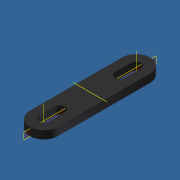
# Autodesk Inventor part: clamp
Saved by Autodesk Inventor 2014 SP2 (Build 180246200, 246)
## iProperties
Created: 2015-02-01
Part Number: clamp
Material: ABS-Kunststoff - Schwarz
Document SubType Name: Modeling
Designer: 4ndreas
Density: 1.06 g/cm^3
Appearance: Glatt - weiß(2)
Author: 4ndreas
Autodesk Inventor part; units mm, degrees
ref_plane "YZ Plane" through (0, 0, 0) normal (1, 0, 0) x (0, 1, 0)
ref_plane "XZ Plane" through (0, 0, 0) normal (0, 1, 0) x (-1, 0, 0)
ref_plane "XY Plane" through (0, 0, 0) normal (0, 0, 1) x (1, 0, 0)
sketch "Skizze1" plane through (0, 0, 0) normal (0, 0, 1) x (1, 0, 0)
  arc A0 (-9.8094, 24.1784) -> (-25.5, 32.4636) centre (-25.5, 13.4636) ccw projected
  spline S0 degree 3 poles (-9.5246, 24.4295) (-9.5947, 24.3508) (-9.6913, 24.2673) (-9.8094, 24.1784) knots -3.5231 -3.5231 -3.5231 -3.5231 -3.387334 -3.387334 -3.387334 -3.387334 projected
  spline S1 degree 3 poles (-5.9203, 24.7286) (-7.1316, 24.6664) (-8.3377, 24.569) (-9.5246, 24.4295) knots -0.358998 -0.358998 -0.358998 -0.358998 -0.000488 -0.000488 -0.000488 -0.000488 projected
  spline S2 degree 3 poles (5.7288, 24.4412) (3.4836, 24.6353) (1.2371, 24.7655) (-2.6308, 24.8325) (-4.2803, 24.8128) (-5.9203, 24.7286) knots -1.514962 -1.514962 -1.514962 -1.514962 -0.844371 -0.844371 -0.358998 -0.358998 -0.358998 -0.358998 projected
  spline S3 degree 3 poles (8.0901, 24.2144) (7.3033, 24.2971) (6.5161, 24.3731) (5.7288, 24.4412) knots -1.750108 -1.750108 -1.750108 -1.750108 -1.514962 -1.514962 -1.514962 -1.514962 projected
  spline S4 degree 3 poles (8.0901, 2.7128) (8.324, 3.0878) (8.9082, 3.5361) (10.1578, 4.5908) (10.8258, 5.1897) (11.6918, 6.3753) (11.9647, 6.883) (12.3113, 8.0997) (12.28, 8.311) (12.28, 12.4461) (12.28, 15.0004) (12.28, 17.8437) (12.2842, 18.1327) (12.2772, 18.5532) (12.2692, 18.684) (12.1997, 19.3209) (12.0468, 19.8567) (11.3337, 21.1434) (10.7675, 21.7557) (9.5317, 22.8964) (8.8596, 23.394) (8.2868, 23.9543) (8.1689, 24.0882) (8.0901, 24.2144) knots -2.176074 -2.176074 -2.176074 -2.176074 -1.773424 -1.773424 -1.41219 -1.41219 -1.17714 -1.17714 -0.899589 -0.899589 -0.451124 -0.451124 -0.400379 -0.400379 -0.377291 -0.377291 -0.287848 -0.287848 -0.17573 -0.17573 -0.044638 -0.044638 0 0 0 0 projected
  spline S5 degree 3 poles (5.7288, 2.4861) (6.516, 2.5542) (7.3031, 2.6301) (8.0901, 2.7128) knots -0.237402 -0.237402 -0.237402 -0.237402 0 0 0 0 projected
  spline S6 degree 3 poles (-5.9203, 2.1987) (-3.7153, 2.0854) (-1.4799, 2.0879) (2.3946, 2.2331) (4.062, 2.342) (5.7288, 2.4861) knots -1.404313 -1.404313 -1.404313 -1.404313 -0.740078 -0.740078 -0.237402 -0.237402 -0.237402 -0.237402 projected
  spline S7 degree 3 poles (-9.5247, 2.4977) (-8.5957, 2.3885) (-7.6099, 2.3) (-6.3513, 2.2219) (-6.1359, 2.2098) (-5.9203, 2.1987) knots -1.784609 -1.784609 -1.784609 -1.784609 -1.469283 -1.469283 -1.404313 -1.404313 -1.404313 -1.404313 projected
  spline S8 degree 3 poles (-9.8094, 2.7489) (-9.6931, 2.6614) (-9.5956, 2.5775) (-9.5247, 2.4977) knots -0.032025 -0.032025 -0.032025 -0.032025 0 0 0 0 projected
  arc A1 (-25.5, -5.5364) -> (-9.8094, 2.7489) centre (-25.5, 13.4636) ccw projected
  line L0 (-9, -5.5364) -> (-25.5, -5.5364) projected
  arc A2 (-7, -7.5364) -> (-9, -5.5364) centre (-9, -7.5364) ccw projected
  line L1 (-7, -7.5364) -> (-7, -9.5364) projected
  arc A3 (-7, -9.5364) -> (-3.4817, -15.6091) centre (0, -9.5364) ccw projected
  line L2 (-3.4817, -15.6091) -> (15.2239, -26.3335) projected
  spline S9 degree 3 poles (15.2239, -26.3335) (17.8166, -26.541) (20.4738, -26.7661) (23.158, -27.0105) knots -4.735814 -4.735814 -4.735814 -4.735814 -3.935681 -3.935681 -3.935681 -3.935681 projected
  spline S10 degree 3 poles (23.158, -27.0105) (27.9304, -27.4451) (32.7882, -27.9415) (37.5208, -28.5102) knots -3.935681 -3.935681 -3.935681 -3.935681 -2.513113 -2.513113 -2.513113 -2.513113 projected
  spline S11 degree 3 poles (37.5208, -28.5102) (38.7326, -28.6558) (39.9362, -28.8061) (44.0796, -29.3451) (47.0402, -29.7682) (50, -30.2427) knots -2.513113 -2.513113 -2.513113 -2.513113 -2.148859 -2.148859 -1.24681 -1.24681 -1.24681 -1.24681 projected
  spline S12 degree 3 poles (56.3465, -31.3443) (54.2358, -30.9481) (52.1208, -30.5826) (50, -30.2427) knots 0.602362 0.602362 0.602362 0.602362 1.248335 1.248335 1.248335 1.248335 projected
  spline S13 degree 3 poles (62.241, -32.537) (60.2791, -32.11) (58.3146, -31.7138) (56.3465, -31.3443) knots 0 0 0 0 0.602362 0.602362 0.602362 0.602362 projected
  spline S14 degree 3 poles (70, -33.3784) (68.7046, -33.3784) (67.4128, -33.3082) (64.8217, -33.0283) (63.5264, -32.8168) (62.241, -32.537) knots 0 0 0 0 0.388621 0.388621 0.78344 0.78344 0.78344 0.78344 projected
  spline S15 degree 3 poles (73.7911, -33.2247) (72.5308, -33.327) (71.2661, -33.3784) (70, -33.3784) knots 14.377982 14.377982 14.377982 14.377982 14.757802 14.757802 14.757802 14.757802 projected
  spline S16 degree 3 poles (73.7911, 60.152) (78.5926, 59.7621) (83.3131, 58.6332) (93.4264, 54.4829) (98.563, 51.0872) (107.2455, 42.5179) (110.7083, 37.4263) (115.4874, 26.2024) (116.7579, 20.1773) (116.918, 7.9793) (115.806, 1.923) (111.3231, -9.4225) (107.9951, -14.6032) (99.5405, -23.3974) (94.4948, -26.9267) (85.9433, -30.7012) (82.8435, -31.7002) (77.726, -32.7793) (75.764, -33.0645) (73.7911, -33.2247) knots 0.380169 0.380169 0.380169 0.380169 1.829857 1.829857 3.659713 3.659713 5.48957 5.48957 7.319427 7.319427 9.149284 9.149284 10.97914 10.97914 12.808997 12.808997 13.783399 13.783399 14.377982 14.377982 14.377982 14.377982 projected
  spline S17 degree 3 poles (70, 60.3056) (71.2672, 60.3056) (72.5319, 60.2542) (73.7911, 60.152) knots 0 0 0 0 0.380169 0.380169 0.380169 0.380169 projected
  spline S18 degree 3 poles (62.241, 59.4643) (63.5284, 59.7445) (64.8258, 59.9562) (67.4171, 60.2358) (68.7068, 60.3056) (70, 60.3056) knots 0 0 0 0 0.395273 0.395273 0.783108 0.783108 0.783108 0.783108 projected
  spline S19 degree 3 poles (56.348, 58.2721) (58.3166, 58.6416) (60.281, 59.0377) (62.241, 59.4643) knots 0.694959 0.694959 0.694959 0.694959 1.295729 1.295729 1.295729 1.295729 projected
  spline S20 degree 3 poles (50, 57.1701) (52.1206, 57.5101) (54.2367, 57.8758) (56.348, 58.2721) knots 0.050632 0.050632 0.050632 0.050632 0.694959 0.694959 0.694959 0.694959 projected
  spline S21 degree 3 poles (50, 57.1701) (47.8223, 56.8209) (45.643, 56.4993) (41.5192, 55.9333) (39.5312, 55.6787) (37.5208, 55.4371) knots -7.681277 -7.681277 -7.681277 -7.681277 -7.051754 -7.051754 -6.488882 -6.488882 -6.488882 -6.488882 projected
  spline S22 degree 3 poles (37.5208, 55.4371) (32.7747, 54.867) (27.9035, 54.3706) (23.158, 53.9385) knots -6.488882 -6.488882 -6.488882 -6.488882 -5.160068 -5.160068 -5.160068 -5.160068 projected
  spline S23 degree 3 poles (23.158, 53.9385) (20.4571, 53.6926) (17.797, 53.4672) (15.2237, 53.2609) knots -5.160068 -5.160068 -5.160068 -5.160068 -4.403779 -4.403779 -4.403779 -4.403779 projected
  line L3 (15.2237, 53.2609) -> (-3.4817, 42.5363) projected
  arc A4 (-3.4817, 42.5363) -> (-7, 36.4636) centre (0, 36.4636) ccw projected
  line L4 (-7, 36.4636) -> (-7, 34.4636) projected
  arc A5 (-9, 32.4636) -> (-7, 34.4636) centre (-9, 34.4636) ccw projected
  line L5 (-25.5, 32.4636) -> (-9, 32.4636) projected
  circle A6 centre (70, 13.4636) radius 11.1 projected
  line L6 (58.1754, -1.5364) -> (56.5877, 1.2136) projected
  line L7 (56.5877, -4.2864) -> (58.1754, -1.5364) projected
  line L8 (53.4123, -4.2864) -> (56.5877, -4.2864) projected
  line L9 (51.8246, -1.5364) -> (53.4123, -4.2864) projected
  line L10 (53.4123, 1.2136) -> (51.8246, -1.5364) projected
  line L11 (56.5877, 1.2136) -> (53.4123, 1.2136) projected
  line L12 (56.5877, 25.7136) -> (58.1754, 28.4636) projected
  line L13 (53.4123, 25.7136) -> (56.5877, 25.7136) projected
  line L14 (51.8246, 28.4636) -> (53.4123, 25.7136) projected
  line L15 (53.4123, 31.2136) -> (51.8246, 28.4636) projected
  line L16 (56.5877, 31.2136) -> (53.4123, 31.2136) projected
  line L17 (58.1754, 28.4636) -> (56.5877, 31.2136) projected
  arc A7 (91, 7.9636) -> (99, 7.9636) centre (95, 7.9636) ccw projected
  line L18 (91, 7.9636) -> (91, 18.9636) projected
  arc A8 (99, 18.9636) -> (91, 18.9636) centre (95, 18.9636) ccw projected
  line L19 (99, 18.9636) -> (99, 7.9636) projected
  line L20 (88.1754, 28.4636) -> (86.5877, 31.2136) projected
  line L21 (86.5877, 25.7136) -> (88.1754, 28.4636) projected
  line L22 (83.4123, 25.7136) -> (86.5877, 25.7136) projected
  line L23 (81.8246, 28.4636) -> (83.4123, 25.7136) projected
  line L24 (83.4123, 31.2136) -> (81.8246, 28.4636) projected
  line L25 (86.5877, 31.2136) -> (83.4123, 31.2136) projected
  line L26 (86.5877, -4.2864) -> (88.1754, -1.5364) projected
  line L27 (83.4123, -4.2864) -> (86.5877, -4.2864) projected
  line L28 (81.8246, -1.5364) -> (83.4123, -4.2864) projected
  line L29 (83.4123, 1.2136) -> (81.8246, -1.5364) projected
  line L30 (86.5877, 1.2136) -> (83.4123, 1.2136) projected
  line L31 (88.1754, -1.5364) -> (86.5877, 1.2136) projected
  line L32 (2.5, -9.5364) -> (2.5, -1.5364) projected
  arc A9 (-2.5, -9.5364) -> (2.5, -9.5364) centre (0, -9.5364) ccw projected
  line L33 (-2.5, -9.5364) -> (-2.5, -1.5364) projected
  arc A10 (2.5, -1.5364) -> (-2.5, -1.5364) centre (0, -1.5364) ccw projected
  line L34 (2.5, 36.4636) -> (2.5, 28.4636) projected
  arc A11 (-2.5, 28.4636) -> (2.5, 28.4636) centre (0, 28.4636) ccw projected
  line L35 (-2.5, 36.4636) -> (-2.5, 28.4636) projected
  arc A12 (2.5, 36.4636) -> (-2.5, 36.4636) centre (0, 36.4636) ccw projected
  line L36 (0, 36.4636) -> (0, -9.5364) construction
  line L37 (-7, 36.4636) -> (-7, -9.5364)
  line L38 (7, -9.5364) -> (7, 36.4636)
  arc A13 (7, 36.4636) -> (-7, 36.4636) centre (0, 36.4636) ccw
  arc A14 (-7, -9.5364) -> (7, -9.5364) centre (0, -9.5364) ccw
  point P0 (0, 0)
  point P1 (0, 13.4636)
  constraints: 8 end point, 6 tangent, 4 point on circle, 2 centre point, 2 parallel, 1 midpoint
extrude "Extrusion1" add sketch "Skizze1" along normal blind 4 contours L37 L4 A4 A13 L38 S3 S2 S1 | S1 S2 S3 L38 S5 S6 S7 L37 | S7 S6 S5 L38 A14 A3 L1 L37
ref_plane "Arbeitsebene1" through (0, -9.5364, 0) normal (-1, 0, 0) x (0, 0, 1)
sketch "Skizze2" plane through (0, 0, 0) normal (0, 0, -1) x (-1, 0, 0)
  arc A0 (7, 36.4636) -> (-7, 36.4636) centre (0, 36.4636) ccw projected
  line L0 (-7, -9.5364) -> (-7, 36.4636) projected
  arc A1 (-7, -9.5364) -> (7, -9.5364) centre (0, -9.5364) ccw projected
  line L1 (0, 36.4636) -> (0, -9.5364) construction
  point P0 (0, 0)
  point P1 (0, 13.4636)
  constraints: 2 end point, 1 midpoint, 1 parallel
hole "Bohrung1" at (0, 13.4636, 0) direction (0, 0, 1) diameter 4 end through all
